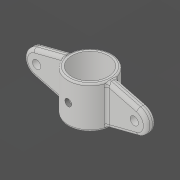
# Autodesk Inventor part: LM51-7
Saved by Autodesk Inventor 2021 (Build 250183000, 183)
## iProperties
Created: 2020-04-23
Part Number: LM51-7
Material: Generic
Document SubType Name: Modeling
Designer: Hannah
Density: 1 g/cm^3
Appearance: Default
Author: Hannah
Autodesk Inventor part; units mm, degrees
ref_plane "YZ Plane" through (0, 0, 0) normal (1, 0, 0) x (0, 1, 0)
ref_plane "XZ Plane" through (0, 0, 0) normal (0, 1, 0) x (-1, 0, 0)
ref_plane "XY Plane" through (0, 0, 0) normal (0, 0, 1) x (1, 0, 0)
sketch "Sketch2" plane through (0, 0, 0) normal (0, 1, 0) x (-1, 0, 0)
  circle A0 centre (0, 0) radius 22
  circle A1 centre (0, 0) radius 26.5
  dimension "d5" = 44
  dimension "d6" = 53
  constraints: 2 centre point, 2 coincident
  measures "d5" diameter of A0
  measures "d6" diameter of A1
extrude "Extrusion2" add sketch "Sketch2" along normal mid plane 50 contours A0 | A1
extrude "Extrusion3" cut sketch "Sketch2" along normal through all both and the other way through all contours A0
hole "Hole1" at (0, 0, 0) direction (0, 0, 1) diameter 8.376 end through all thread size "M10x1.5" class "6H" standard "ISO Metric profile"
sketch "Sketch3" plane through (0, 0, 0) normal (0, 0, 1) x (1, 0, 0)
  circle A0 centre (59, 0) radius 5
  arc A1 (62.7349, -14.5276) -> (62.7349, 14.5276) centre (59, 0) ccw
  line L0 (22, 25) -> (62.7349, 14.5276)
  line L1 (62.7349, -14.5276) -> (22, -25)
  line L2 (0, -32.9) -> (0, 32.9) projected
  line L3 (22, -25) -> (22, 25) projected
  circle A2 centre (-59, 0) radius 5
  arc A3 (-62.7349, 14.5276) -> (-62.7349, -14.5276) centre (-59, 0) ccw
  line L4 (-22, 25) -> (-62.7349, 14.5276)
  line L5 (-62.7349, -14.5276) -> (-22, -25)
  line L6 (-22, -25) -> (-22, 25)
  point P0 (0, 0)
  dimension "d36" = 10
  dimension "d37" = 15
  dimension "d40" = 59
  constraints: 10 end point, 6 symmetric about line, 4 centre point, 4 point on circle, 2 coincident, 2 tangent, 1 equal length, 2 other
  measures "d36" diameter of A0
  measures "d37" radius of A1
  measures "d40" distance from line of L2 A0.centre
extrude "Extrusion5" add sketch "Sketch3" along normal mid plane 11
fillet "Fillet2" radius 4 12 edges at (74, 0, 5.5) (44.3289, -19.2595, 5.5) (44.3289, 19.2595, 5.5) (74, 0, -5.5) (44.3289, -19.2595, -5.5) (44.3289, 19.2595, -5.5) (-74, 0, 5.5) (-44.3289, -19.2595, 5.5) (-44.3289, 19.2595, 5.5) (-74, 0, -5.5) (-44.3289, -19.2595, -5.5) (-44.3289, 19.2595, -5.5)
fillet "Fillet2" radius 2 2 edges at (26.5, 25, 0) (26.5, -25, 0)
fillet "Fillet3" radius 4 26 edges at (25.923, 0, 5.5) (25.9942, 21.5259, 5.1529) (26.2301, 23.6683, 2.8549) (26.2871, 23.8978, -0.0001) (26.2301, 23.6683, -2.8549) (25.9942, 21.5259, -5.1529) (25.923, 0, -5.5) (25.9942, -21.5259, -5.1529) (26.2301, -23.6683, -2.8549) (26.2871, -23.8978, -0.0001) (26.2301, -23.6683, 2.8549) (25.9942, -21.5259, 5.1529) (-25.9942, 21.5259, 5.1529) (-26.2301, 23.6683, 2.8549) (-26.2748, 23.901, -0.7505) (-26.2748, 23.901, 0.7505) (-26.2301, 23.6683, -2.8549) (-25.9942, 21.5259, -5.1529) (-25.923, 0, -5.5) (-25.9942, -21.5259, -5.1529) (-26.2301, -23.6683, -2.8549) (-26.2748, -23.901, -0.7505) (-26.2748, -23.901, 0.7505) (-26.2301, -23.6683, 2.8549) (-25.9942, -21.5259, 5.1529) (-25.923, 0, 5.5)
body "Solid1"
